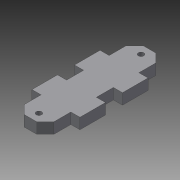
# Autodesk Inventor part: Air2D_Bottom
Saved by Autodesk Inventor 2014 (Build 180170000, 170)
## iProperties
Created: 2014-09-30
Part Number: Air2D_Bottom
Material: Generic
Document SubType Name: Modeling
Designer: ThatOtherGuy
Density: 1 g/cm^3
Appearance: Default
Author: ThatOtherGuy
Autodesk Inventor part; units mm, degrees
ref_plane "YZ Plane" through (0, 0, 0) normal (1, 0, 0) x (0, 1, 0)
ref_plane "XZ Plane" through (0, 0, 0) normal (0, 1, 0) x (-1, 0, 0)
ref_plane "XY Plane" through (0, 0, 0) normal (0, 0, 1) x (1, 0, 0)
sketch "Sketch1" plane through (0, 0, 0) normal (0, 0, 1) x (1, 0, 0)
  line L0 (0, 0) -> (17.5, 0)
  line L1 (17.5, 0) -> (17.5, 70)
  line L2 (17.5, 70) -> (0, 70)
  line L3 (0, 70) -> (0, 0)
  line L4 (0, 55) -> (-5.731, 55)
  line L5 (-5.731, 55) -> (-5.731, 40)
  line L6 (-5.731, 40) -> (0, 40)
  line L7 (0, 40) -> (0, 55)
  line L8 (0, 30) -> (-5.731, 30)
  line L9 (-5.731, 30) -> (-5.731, 15)
  line L10 (-5.731, 15) -> (0, 15)
  line L11 (0, 15) -> (0, 30)
  circle A0 centre (8.75, 65) radius 1.6
  circle A1 centre (8.75, 5) radius 1.6
  line L12 (17.5, 55) -> (23.231, 55)
  line L13 (23.231, 55) -> (23.231, 40)
  line L14 (23.231, 40) -> (17.5, 40)
  line L15 (17.5, 40) -> (17.5, 55)
  line L16 (17.5, 30) -> (23.231, 30)
  line L17 (23.231, 30) -> (23.231, 15)
  line L18 (23.231, 15) -> (17.5, 15)
  line L19 (17.5, 15) -> (17.5, 30)
  point P0 (8.75, 70)
  dimension "d0" = 17.5
  dimension "d1" = 70
  dimension "d2" = 15
  dimension "d3" = 5.731
  dimension "d4" = 10
  dimension "d5" = 15
  dimension "d6" = 15
  dimension "d7" = 3.2
  dimension "d8" = 5
  dimension "d9" = 5
  constraints: 40 end point, 10 parallel, 6 equal length, 5 horizontal, 5 perpendicular, 4 point on line, 2 centre point, 2 collinear, 2 vertical alignment, 1 equal radius, 1 midpoint
  measures "d0" distance of L0.start L0.end
  measures "d1" distance of L2.end L0.start
  measures "d2" distance of L4.end L5.end
  measures "d3" distance of L8.start L8.end
  measures "d4" distance between parallel lines of L6 L8
  measures "d5" distance between parallel lines of L0 L10
  measures "d6" distance between parallel lines of L2 L4
  measures "d7" diameter of A0
  measures "d8" distance from line of L0 A1.centre
  measures "d9" distance from line of A0.centre L2
extrude "Extrusion1" add sketch "Sketch1" along normal blind 6.731
chamfer "Chamfer1" distance 5 angle 45 4 edges at (0, 70, 3.3655) (17.5, 70, 3.3655) (0, 0, 3.3655) (17.5, 0, 3.3655)
equation "\"d5\" = d6"
equation "\"d9\" = d8"
equation "\"d10\" = THICKB"
equation "\"THICKA\" = 3.175"
equation "\"THICKB\" = 6.731"
equation "\"THICKC\" = 12.7"
equation "\"MAGDIA\" = 9.5"
equation "\"BALLDIA\" = 12"
body "Solid1"
